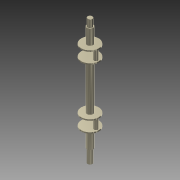
# Autodesk Inventor part: 砂轮架带动曲轴
Saved by Autodesk Inventor 2015 (Build 190159000, 159)
## iProperties
Created: 2017-05-17
Part Number: 砂轮架带动曲轴
Material: 常规
Document SubType Name: Modeling
Designer: Administrator
Density: 1 g/cm^3
Appearance: 镍
Author: Administrator
Autodesk Inventor part; units mm, degrees
ref_plane "YZ Plane" through (0, 0, 0) normal (1, 0, 0) x (0, 1, 0)
ref_plane "XZ Plane" through (0, 0, 0) normal (0, 1, 0) x (-1, 0, 0)
ref_plane "XY Plane" through (0, 0, 0) normal (0, 0, 1) x (1, 0, 0)
sketch "草图1" plane through (0, 0, 0) normal (0, 0, 1) x (1, 0, 0)
  circle A0 centre (0, 0) radius 12.5
  dimension "d0" = 25
  constraints: 1 centre point, 1 coincident
  measures "d0" diameter of A0
extrude "拉伸1" add sketch "草图1" along normal blind 103
sketch "草图2" plane through (0, 0, 103) normal (0, 0, 1) x (1, 0, 0)
  circle A0 centre (0, 0) radius 35
  dimension "d3" = 70
  constraints: 1 centre point, 1 coincident
  measures "d3" diameter of A0
extrude "拉伸2" add sketch "草图2" along normal blind 5
sketch "草图3" plane through (0, 0, 108) normal (0, 0, 1) x (1, 0, 0)
  circle A0 centre (24, 0) radius 7.5
  line L0 (0, 0) -> (4.085, 0)
  dimension "d6" = 15
  dimension "d7" = 4.085
  dimension "d8" = 24
  constraints: 2 end point, 1 centre point, 1 horizontal, 1 point on line
  measures "d6" diameter of A0
  measures "d7" distance of L0.start L0.end
  measures "d8" distance of L0.start A0.centre
extrude "拉伸3" add sketch "草图3" along normal blind 40
sketch "草图4" plane through (24, 0, 148) normal (0, 0, 1) x (1, 0, 0)
  circle A0 centre (-24, 0) radius 35
  circle A1 centre (-24, 0) radius 35 projected
  dimension "d11" = 70
  constraints: 1 centre point, 1 concentric
  measures "d11" diameter of A0
extrude "拉伸4" add sketch "草图4" along normal blind 5
sketch "草图5" plane through (0, 0, 153) normal (0, 0, 1) x (1, 0, 0)
  circle A0 centre (0, 0) radius 12.5
  dimension "d14" = 25
  constraints: 1 centre point, 1 coincident
  measures "d14" diameter of A0
extrude "拉伸5" add sketch "草图5" along normal blind 190
sketch "草图6" plane through (0, 0, 343) normal (0, 0, 1) x (1, 0, 0)
  circle A0 centre (0, 0) radius 35
  dimension "d17" = 70
  constraints: 1 centre point, 1 coincident
  measures "d17" diameter of A0
extrude "拉伸6" add sketch "草图6" along normal blind 5
sketch "草图7" plane through (0, 0, 348) normal (0, 0, 1) x (1, 0, 0)
  circle A0 centre (24, 0) radius 7.5
  circle A1 centre (24, 0) radius 7.5 projected
  point P0 (0, 0)
  dimension "d20" = 15
  constraints: 1 centre point, 1 concentric
  measures "d20" diameter of A0
extrude "拉伸7" add sketch "草图7" along normal blind 40
sketch "草图8" plane through (24, 0, 388) normal (0, 0, 1) x (1, 0, 0)
  circle A0 centre (-24, 0) radius 12.5 projected
  circle A1 centre (-24, 0) radius 35
  dimension "d23" = 70
  constraints: 1 centre point, 1 coincident
  measures "d23" diameter of A1
extrude "拉伸8" add sketch "草图8" along normal blind 5 contours A0 | A1
sketch "草图9" plane through (0, 0, 393) normal (0, 0, 1) x (1, 0, 0)
  circle A0 centre (0, 0) radius 12.5
  dimension "d26" = 25
  constraints: 1 centre point, 1 coincident
  measures "d26" diameter of A0
extrude "拉伸9" add sketch "草图9" along normal blind 90
sketch "草图10" plane through (0, 0, 483) normal (0, 0, 1) x (1, 0, 0)
  circle A0 centre (0, 0) radius 10
  circle A1 centre (0, 0) radius 12.5
  dimension "d32" = 20
  dimension "d33" = 25
  constraints: 2 centre point, 2 coincident
  measures "d32" diameter of A0
  measures "d33" diameter of A1
extrude "拉伸10" cut sketch "草图10" against normal blind 30
chamfer "倒角2" distance 1 angle 45 1 edges at (-10, 0, 483)
sketch "草图11" plane through (0, 0, 0) normal (0, 0, -1) x (-1, 0, 0)
  circle A0 centre (0, 0) radius 10
  circle A1 centre (0, 0) radius 12.5
  dimension "d39" = 20
  dimension "d40" = 25
  constraints: 2 centre point, 2 coincident
  measures "d39" diameter of A0
  measures "d40" diameter of A1
extrude "拉伸11" cut sketch "草图11" against normal blind 30
sketch "草图12" plane through (0, 0, 0) normal (0, 0, -1) x (-1, 0, 0)
  circle A0 centre (0, 0) radius 10
  dimension "d43" = 20
  constraints: 1 centre point, 1 coincident
  measures "d43" diameter of A0
extrude "拉伸12" add sketch "草图12" along normal blind 22
